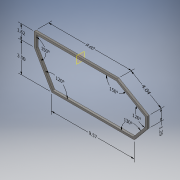
# Autodesk Inventor part: Cabin Frame
Saved by Autodesk Inventor 2019 (Build 230136000, 136)
## iProperties
Created: 2019-08-30
Part Number: Cabin Frame
Material: Steel, Mild
Document SubType Name: Modeling
Designer: DIBYOJYOTI
Density: 7.85 g/cm^3
Appearance: Semi-Polished
Author: DIBYOJYOTI
Autodesk Inventor part; units mm, degrees
ref_plane "YZ Plane" through (0, 0, 0) normal (1, 0, 0) x (0, 1, 0)
ref_plane "XZ Plane" through (0, 0, 0) normal (0, 1, 0) x (-1, 0, 0)
ref_plane "XY Plane" through (0, 0, 0) normal (0, 0, 1) x (1, 0, 0)
derived "Cabin Wall.ipt"
ref_plane "Work Plane1" through (50, 117, -4) normal (1, 0, 0) x (0, 1, 0)
sketch "Sketch2" plane through (50, 117, -4) normal (1, 0, 0) x (0, 1, 0)
  line L0 (-3, 3) -> (3, 3)
  line L1 (3, 3) -> (3, -3)
  line L2 (3, -3) -> (-3, -3)
  line L3 (-3, -3) -> (-3, 3)
  line L4 (-3, 3) -> (3, -3) construction
  line L5 (3, 3) -> (-3, -3) construction
  point P0 (-117, 4)
  point P1 (0, 0)
  dimension "d1" = 6
  dimension "d2" = 6
  constraints: 12 end point, 2 midpoint, 2 parallel, 1 horizontal, 1 perpendicular
  measures "d1" distance of L1.end L2.end
  measures "d2" distance of L0.end L1.end
sketch "Sketch3" plane through (110, 117, -4) normal (0, 0, -1) x (-1, 0, 0)
  line L0 (0, 0) -> (-50, 0)
  line L1 (0, 0) -> (50, 0) construction
  line L2 (-50, 0) -> (-136.6025, -50)
  line L3 (-50, 0) -> (50, 0) construction
  line L4 (-136.6025, -50) -> (-136.6025, -80)
  line L5 (-50, -124) -> (110, -124)
  line L6 (-50, -124) -> (-100, -124)
  line L7 (-100, -124) -> (-136.6025, -80)
  line L8 (110, -124) -> (140, -124)
  line L9 (140, -124) -> (190, -37.3975)
  line L10 (60, 0) -> (0, 0)
  line L11 (0, 0) -> (60, 0)
  line L12 (60, 0) -> (190, 0)
  line L13 (190, 0) -> (190, -37.3975)
  point P0 (110, -117)
  constraints: 28 end point
sweep "Sweep1" add profiles "Sketch2" path "Sketch3" path curves L10 L0 L2 L4 L7 L6 L5 L8 L9 L13 L12
body "Solid1"
